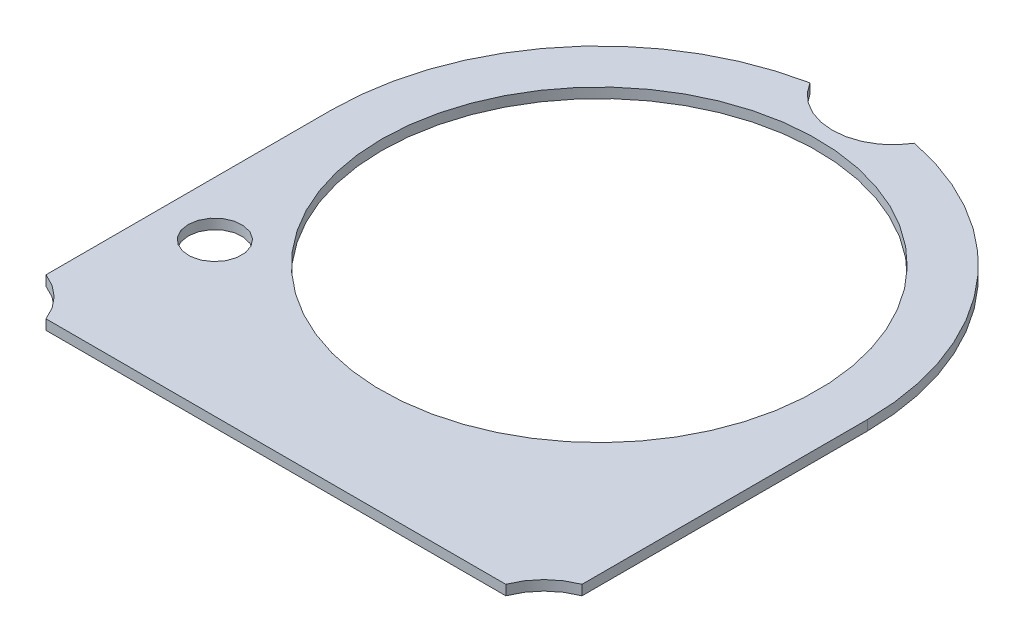
# Autodesk Inventor part: pcb
Saved by Autodesk Inventor 2026.2 (Build 302298000, 298)
## iProperties
Created: 2026-04-07
Part Number: pcb
Material: Generic
Document SubType Name: Modeling
Designer: Tathagata Sikdar
Density: 1 g/cm^3
Appearance: Green Polished
Author: Tathagata Sikdar
Autodesk Inventor part; units mm, degrees
ref_plane "YZ Plane" through (0, 0, 0) normal (1, 0, 0) x (0, 1, 0)
ref_plane "XZ Plane" through (0, 0, 0) normal (0, 1, 0) x (-1, 0, 0)
ref_plane "XY Plane" through (0, 0, 0) normal (0, 0, 1) x (1, 0, 0)
ref_plane "Work Plane1" through (-51.7969, 23.5104, -145.9222) normal (0, 1, 0) x (-1, 0, 0)
sketch "Sketch1" plane through (-51.7969, 23.5104, -145.9222) normal (0, 1, 0) x (-1, 0, 0)
  circle A0 centre (64.1421, 42.8631) radius 8 projected
  circle A1 centre (0, -8.3092) radius 65.3144 projected
  line L0 (80.3944, -8.3092) -> (80.3944, 77.2593) projected
  arc A2 (68.9502, 88.7036) -> (80.3944, 77.2593) centre (87.3944, 95.7036) ccw projected
  line L1 (68.9502, 88.7036) -> (-68.9502, 88.7036) projected
  arc A3 (-80.3944, 77.2593) -> (-68.9502, 88.7036) centre (-87.3944, 95.7036) ccw projected
  line L2 (-80.3944, 77.2593) -> (-80.3944, -8.3092) projected
  arc A4 (-80.3944, -8.3092) -> (-15.6866, -87.1584) centre (0, -8.3092) ccw projected
  arc A5 (15.6866, -87.1584) -> (-15.6866, -87.1584) centre (0, -96.4205) ccw projected
  arc A6 (15.6866, -87.1584) -> (80.3944, -8.3092) centre (0, -8.3092) ccw projected
  point P0 (-51.7969, 145.9222)
extrude "Extrusion1" add sketch "Sketch1" along normal blind 3
body "Solid1"
